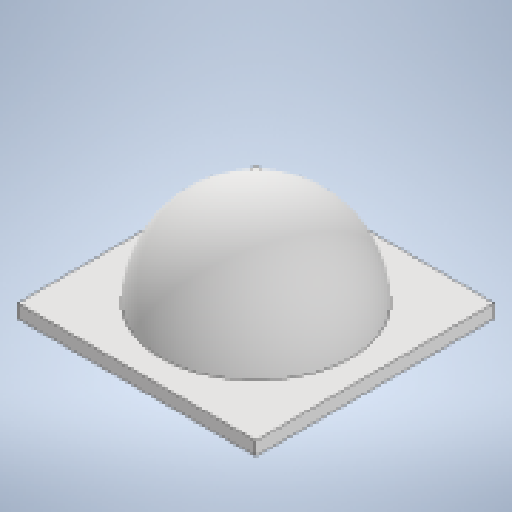
# Autodesk Inventor part: 50w led
Saved by Autodesk Inventor 2025 (Build 290162000, 162)
## iProperties
Created: 2025-08-17
Part Number: 50w led
Material: 一般
Document SubType Name: Modeling
Designer: gavin
Density: 1 g/cm^3
Appearance: 預設
Author: gavin
Autodesk Inventor part; units mm, degrees
ref_plane "YZ Plane" through (0, 0, 0) normal (1, 0, 0) x (0, 1, 0)
ref_plane "XZ Plane" through (0, 0, 0) normal (0, 1, 0) x (-1, 0, 0)
ref_plane "XY Plane" through (0, 0, 0) normal (0, 0, 1) x (1, 0, 0)
sketch "草圖1" plane through (0, 0, 0) normal (0, 1, 0) x (-1, 0, 0)
  line L0 (-14, 14) -> (14, 14)
  line L1 (14, 14) -> (14, -14)
  line L2 (14, -14) -> (-14, -14)
  line L3 (-14, -14) -> (-14, 14)
  line L4 (-14, 14) -> (14, -14) construction
  line L5 (14, 14) -> (-14, -14) construction
  point P0 (0, 0)
  dimension "d0" = 28
  dimension "d1" = 28
  constraints: 12 end point, 2 midpoint, 2 parallel, 1 horizontal, 1 perpendicular
  measures "d0" distance of L1.end L2.end
  measures "d1" distance of L0.end L1.end
extrude "擠出1" add sketch "草圖1" along normal blind 1.6
sketch "草圖2" plane through (0, 0, 0) normal (1, 0, 0) x (0, 1, 0)
  line L0 (1.6, 14) -> (1.6, -14) projected
  circle A0 centre (1.6, 0) radius 11.175
  line L1 (12.775, 0) -> (1.6, 0)
  line L2 (-14.045, 0) -> (17.245, 0) projected
  point P0 (0, 0)
  point P1 (1.6, -11.175)
  dimension "d4" = 22.35
  constraints: 2 end point, 1 horizontal, 1 midpoint, 3 other
revolve "迴轉1" add sketch "草圖2" angle 360 about axis through (0, -10, 0) along (0, 1, 0) picked at (4.0451, -6.9877) contours L1 A0 L0
sketch "草圖3" plane through (0, 1.6, 0) normal (0, 1, 0) x (1, 0, 0)
  circle A0 centre (0, 0) radius 11.175 projected
  line L0 (14, 14) -> (-14, 14) projected
  line L1 (-14, 14) -> (-14, -14) projected
  line L2 (-14, -14) -> (14, -14) projected
  line L3 (14, -14) -> (14, 14) projected
  line L4 (11.175, -11.175) -> (-11.175, -11.175) construction
  line L5 (-11.175, -11.175) -> (-11.175, 11.175) construction
  line L6 (-11.175, 11.175) -> (11.175, 11.175) construction
  line L7 (11.175, 11.175) -> (11.175, -11.175) construction
  line L8 (11.175, -11.175) -> (-11.175, 11.175) construction
  line L9 (-11.175, -11.175) -> (11.175, 11.175) construction
  circle A1 centre (-11.175, 11.175) radius 1.5
  circle A2 centre (11.175, -11.175) radius 1.5
  dimension "d6" = 3
  dimension "d7" = 3
  constraints: 12 end point, 2 centre point, 2 midpoint, 2 parallel, 1 coincident, 1 horizontal, 1 perpendicular
  measures "d6" diameter of A1
  measures "d7" diameter of A2
extrude "擠出2" cut sketch "草圖3" against normal blind 1.6 contours A1 | A2
